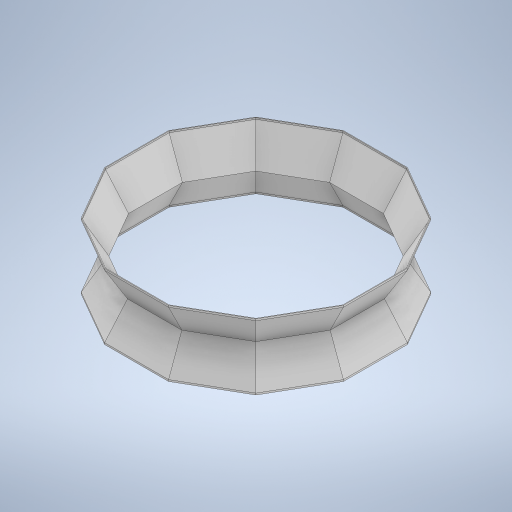
# Autodesk Inventor part: OV-PAM_n_12_standard_1F
Saved by Autodesk Inventor 2024 (Build 280153000, 153)
## iProperties
Created: 2023-08-31
Part Number: OV-PAM_n_12_standard_1F
Material: 일반
Document SubType Name: Modeling
Designer: jsw
Density: 1 g/cm^3
Appearance: 기본값
Author: jsw
Autodesk Inventor part; units mm, degrees
ref_plane "YZ Plane" through (0, 0, 0) normal (1, 0, 0) x (0, 1, 0)
sketch "스케치1" plane through (0, 0, 0) normal (0, 1, 0) x (-1, 0, 0)
  line L0 (-22.8259, 85.1874) -> (22.8259, 85.1874)
  line L1 (22.8259, 85.1874) -> (62.3615, 62.3615)
  line L2 (62.3615, 62.3615) -> (85.1874, 22.8259)
  line L3 (85.1874, 22.8259) -> (85.1874, -22.8259)
  line L4 (85.1874, -22.8259) -> (62.3615, -62.3615)
  line L5 (62.3615, -62.3615) -> (22.8259, -85.1874)
  line L6 (22.8259, -85.1874) -> (-22.8259, -85.1874)
  line L7 (-22.8259, -85.1874) -> (-62.3615, -62.3615)
  line L8 (-62.3615, -62.3615) -> (-85.1874, -22.8259)
  line L9 (-85.1874, -22.8259) -> (-85.1874, 22.8259)
  line L10 (-85.1874, 22.8259) -> (-62.3615, 62.3615)
  line L11 (-62.3615, 62.3615) -> (-22.8259, 85.1874)
  line L12 (22.9867, -85.7874) -> (-22.9867, -85.7874)
  line L13 (-22.9867, -85.7874) -> (-62.8007, -62.8007)
  line L14 (-62.8007, -62.8007) -> (-85.7874, -22.9867)
  line L15 (-85.7874, -22.9867) -> (-85.7874, 22.9867)
  line L16 (-85.7874, 22.9867) -> (-62.8007, 62.8007)
  line L17 (-62.8007, 62.8007) -> (-22.9867, 85.7874)
  line L18 (-22.9867, 85.7874) -> (22.9867, 85.7874)
  line L19 (22.9867, 85.7874) -> (62.8007, 62.8007)
  line L20 (62.8007, 62.8007) -> (85.7874, 22.9867)
  line L21 (85.7874, 22.9867) -> (85.7874, -22.9867)
  line L22 (85.7874, -22.9867) -> (62.8007, -62.8007)
  line L23 (62.8007, -62.8007) -> (22.9867, -85.7874)
  point P0 (0, 0)
  point P1 (0, 0)
  point P2 (0, 0)
  dimension "d1" = 176.385
  dimension "d2" = 0.6
  constraints: 48 end point, 2 coincident, 2 horizontal, 50 other
  measures "d1" distance of L8.end L2.end
  measures "d2" distance between parallel lines of L3 L21
extrude "돌출1" add sketch "스케치1" along normal blind 22.5 contours L0 L1 L2 L3 L4 L5 L6 L7 L8 L9 L10 L11 | L12 L13 L14 L15 L16 L17 L18 L19 L20 L21 L22 L23
ref_plane "작업 평면1" through (62.8007, 0, 62.8007) normal (-0.75, -0.5, -0.4330127) x (0.5, 0, -0.8660254)
sketch "스케치2" plane through (85.7874, 0, 22.9867) normal (0.8660254, 0, 0.5) x (0.5, 0, -0.8660254)
  line L0 (-45.9733, 0) -> (0, 0) projected
  line L1 (0, 0) -> (0, 22.5) projected
  line L2 (-45.9733, 22.5) -> (0, 22.5) projected
  line L3 (-45.9733, 0) -> (-45.9733, 22.5) projected
  line L4 (-45.9733, 0) -> (-85.7874, 0) projected
  line L5 (-45.9733, 0) -> (-84.9445, 22.5)
  line L6 (-45.9733, 22.5) -> (-85.7874, 22.5) projected
  line L7 (0, 0) -> (-1, 22.5)
  line L8 (-45.9733, 22.5) -> (-84.9445, 22.5)
  point P0 (-22.9867, 0)
  point P1 (-85.7874, 27)
  dimension "d6" = 150
  dimension "d7" = 1
  constraints: 6 end point, 2 point on line, 1 collinear
  measures "d6" angle of L5 L0
  measures "d7" distance of L1.end L7.end
extrude "돌출2" cut sketch "스케치2" along normal up to surface contours L3 L2 L7 L0 | L5 L6 L3 surface through (62.8007, 0, 62.8007) normal (-0.75, -0.5, -0.4330127)
pattern_circular "원형 패턴1" count 12 over 360 about axis through (0, -10, 0) along (0, 1, 0) of "돌출2"
sketch "스케치3" plane through (0, 0, 0) normal (0, -1, 0) x (1, 0, 0)
  line L0 (-62.8007, -62.8007) -> (-85.7874, -22.9867) projected
  line L1 (-22.9867, -85.7874) -> (-62.8007, -62.8007) projected
  line L2 (22.9867, -85.7874) -> (-22.9867, -85.7874) projected
  line L3 (62.8007, -62.8007) -> (22.9867, -85.7874) projected
  line L4 (85.7874, -22.9867) -> (62.8007, -62.8007) projected
  line L5 (85.7874, 22.9867) -> (85.7874, -22.9867) projected
  line L6 (62.8007, 62.8007) -> (85.7874, 22.9867) projected
  line L7 (22.9867, 85.7874) -> (62.8007, 62.8007) projected
  line L8 (-22.9867, 85.7874) -> (22.9867, 85.7874) projected
  line L9 (-62.8007, 62.8007) -> (-22.9867, 85.7874) projected
  line L10 (-85.7874, 22.9867) -> (-62.8007, 62.8007) projected
  line L11 (-85.7874, -22.9867) -> (-85.7874, 22.9867) projected
  point P0 (0, 0)
extrude "돌출3" add sketch "스케치3" along normal blind 1.2
ref_plane "작업 평면2" through (0, 22.5, 0) normal (0, 1, 0) x (1, 0, 0)
mirror "미러1" about plane through (0, 22.5, 0) normal (0, 1, 0) of "돌출2", "원형 패턴1", "돌출3", "돌출1"
shell "쉘1" thickness 0.5 removed faces 2 at (7.6622, 46.2, -28.5958) at (-7.6622, -1.2, 28.5958)
